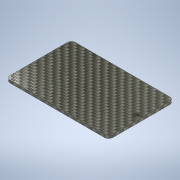
# Autodesk Inventor part: magnet card top
Saved by Autodesk Inventor 2020 (Build 240168000, 168)
## iProperties
Created: 2019-06-07
Part Number: magnet card top
Material: Generic
Document SubType Name: Modeling
Designer: kangh
Density: 1 g/cm^3
Appearance: Carbon Fiber 1
Author: kangh
Autodesk Inventor part; units mm, degrees
ref_plane "YZ Plane" through (0, 0, 0) normal (1, 0, 0) x (0, 1, 0)
ref_plane "XZ Plane" through (0, 0, 0) normal (0, 1, 0) x (-1, 0, 0)
ref_plane "XY Plane" through (0, 0, 0) normal (0, 0, 1) x (1, 0, 0)
sketch "Sketch1" plane through (0, 0, 0) normal (0, 1, 0) x (-1, 0, 0)
  line L0 (0, 0) -> (97.6122, 0)
  line L1 (97.6122, 0) -> (97.6122, 62.1284)
  line L2 (97.6122, 62.1284) -> (0, 62.1284)
  line L3 (0, 62.1284) -> (0, 0)
  line L4 (97.6122, 62.1284) -> (97.6122, 60.1284)
  line L5 (97.6122, 60.1284) -> (74.5998, 60.1284)
  circle A0 centre (74.5998, 60.1284) radius 1
  line L6 (0, 31.0642) -> (4.5, 31.0642)
  circle A1 centre (4.5, 31.0642) radius 2.5
  line L7 (4.5, 31.0642) -> (97.6122, 31.0642)
  circle A2 centre (74.5998, 2) radius 1
  dimension "d0" = 97.6122
  dimension "d1" = 62.1284
  dimension "d2" = 2
  dimension "d3" = 23.0124
  dimension "d4" = 2
  dimension "d5" = 4.5
  dimension "d6" = 5
  constraints: 16 end point, 3 centre point, 2 coincident, 2 horizontal, 2 midpoint, 2 parallel, 2 perpendicular, 1 point on line, 1 symmetric about line, 1 other
  measures "d0" distance of L2.end L1.end
  measures "d1" distance of L1.end L0.end
  measures "d2" distance of L1.end L4.end
  measures "d3" distance of L4.end L5.end
  measures "d4" diameter of A0
  measures "d5" distance of L6.start L6.end
  measures "d6" diameter of A1
extrude "Extrusion1" add sketch "Sketch1" along normal blind 3 contours L3 L6 A1 L7 L1 L0 | L3 L2 L1 L7 A1 L6
extrude "Extrusion2" add sketch "Sketch1" along normal blind 1 contours A1 L7 L6 | L6 L7 A1 | A0 | A2
fillet "Fillet1" radius 4 4 edges at (-97.6122, 1.5, 62.1284) (-97.6122, 1.5, 0) (0, 1.5, 0) (0, 1.5, 62.1284)
move faces "Move1" translate (0, 0.5, 0) faces at (-63.7415, 0, 20.7095)
body "Solid1"
